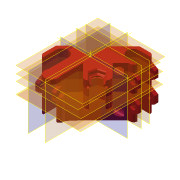
# Autodesk Inventor part: Cycl_carroX
Saved by Autodesk Inventor 2015 SP2 (Build 190223200, 223)
## iProperties
Created: 2015-05-05
Material: Genérico
Document SubType Name: Modeling
Designer: E.Beroiz
Density: 1 g/cm^3
Appearance: Light Red
Description: Cycl_carroX
Author: E.Beroiz
Autodesk Inventor part; units mm, degrees
sketch "Boceto1" plane through (0, 0, 0) normal (0, 0, 1) x (1, 0, 0)
  line L0 (0, 0) -> (0, 20)
  line L1 (0, 20) -> (17.4688, 37.4774)
  line L2 (17.4688, 37.4774) -> (29.4688, 37.4774)
  arc A0 (33.4688, 33.4774) -> (29.4688, 37.4774) centre (29.4688, 33.4774) ccw
  line L3 (33.4688, 33.4774) -> (21.7203, 33.4774)
  arc A1 (21.7203, 33.4774) -> (21.7203, 19.1774) centre (21.7203, 26.3274) ccw
  line L4 (21.7203, 19.1774) -> (33.4688, 19.1774)
  arc A2 (29.4688, 15.1774) -> (33.4688, 19.1774) centre (29.4688, 19.1774) ccw
  line L5 (29.4688, 15.1774) -> (27.2204, 15.1774)
  line L6 (27.2204, 15.1774) -> (18.5336, 6.4864)
  line L7 (18.5336, 6.4864) -> (31.5759, -6.5494)
  arc A3 (31.5778, -14.4125) -> (31.5759, -6.5494) centre (27.6454, -10.4819) ccw
  line L8 (31.5778, -14.4125) -> (23.3026, -6.1413)
  line L9 (23.3026, -6.1413) -> (15.9976, -8.1007)
  line L10 (15.9976, -8.1007) -> (14.0418, -15.4067)
  line L11 (14.0418, -15.4067) -> (22.317, -23.6778)
  arc A4 (15.7833, -23.6794) -> (22.317, -23.6778) centre (19.0494, -20.4118) ccw
  line L12 (15.7833, -23.6794) -> (2.0762, -9.9791)
  line L13 (2.0762, -9.9791) -> (2.0762, -34.9791)
  arc A5 (-11.2738, -34.9791) -> (2.0762, -34.9791) centre (-4.5988, -38.3988) ccw
  line L14 (-11.2738, -34.9791) -> (-11.2738, -13.0246)
  arc A6 (-11.2738, -13.0246) -> (-25.5738, -13.0246) centre (-18.4238, -13.0246) ccw
  line L15 (-25.5738, -13.0246) -> (-25.5738, -26.5746)
  arc A7 (-29.5738, -22.5746) -> (-25.5738, -26.5746) centre (-25.5738, -22.5746) ccw
  line L16 (-29.5738, -22.5746) -> (-29.5738, -8.5746)
  line L17 (-29.5738, -8.5746) -> (-21, 0)
  line L18 (-21, 0) -> (0, 0)
  circle A8 centre (21.3255, -13.4245) radius 4 projected
  dimension "d0" = 20
  dimension "d3" = 16
  dimension "d7" = 4
  dimension "d8" = 4
  dimension "d10" = 5.56
  dimension "d11" = 4.62
  dimension "d12" = 13.1
  dimension "d13" = 11.7
  dimension "d14" = 11.7
  dimension "d15" = 24
  dimension "d16" = 24
  dimension "d17" = 120
  dimension "d18" = 0
  dimension "d19" = 25
  dimension "d21" = 7.5
  dimension "d23" = 21
  dimension "d24" = 18
  dimension "d25" = 4
  dimension "d26" = 14.3
  dimension "d97" = 56.215
  dimension "d98" = 7.15
  dimension "d99" = 135.003
  dimension "d100" = 135.014
  dimension "d101" = 11.7485
  dimension "d102" = 2.0762
  dimension "d109" = 6.4864
  dimension "d110" = 6.551
  dimension "d111" = 6.549
  dimension "d115" = 20.5
  dimension "d116" = 19.841
  dimension "d118" = 14.3
  constraints: 38 end point, 16 point on circle, 8 centre point, 8 tangent, 7 parallel, 5 vertical, 3 horizontal alignment, 3 point on line, 2 perpendicular, 2 vertical alignment, 1 equal length, 1 horizontal
  measures "d0" distance of L0.start L0.end
  measures "d3" horizontal distance of L1.end L3.start
  measures "d7" distance between parallel lines of L3 L2
  measures "d8" distance between parallel lines of L5 L4
  measures "d10" distance between parallel lines of L7 L8
  measures "d11" distance from line of L12.start L11
  measures "d12" distance between parallel lines of L11 L8
  measures "d13" distance of L8.start L8.end
  measures "d14" distance of L10.end L11.end
  measures "d15" distance from line of L8.start L6
  measures "d16" distance from line of L11.end L6
  measures "d17" angle of L10 L9
  measures "d18" distance from line of L12.end L6
  measures "d19" distance of L12.end L13.end
  measures "d21" radius of A5
  measures "d23" distance of L17.end L0.start
  measures "d24" vertical distance of L16.end L15.end
  measures "d25" distance between parallel lines of L15 L16
  measures "d26" distance between parallel lines of L15 L14
  measures "d97" distance of A1.centre A6.centre
  measures "d98" radius of A6
  measures "d99" angle of L17 L16
  measures "d100" angle of L0 L1
  measures "d101" distance of L4.start L4.end
  measures "d102" distance from line of L0.start L13
  measures "d109" vertical distance of L6.end L0.start
  measures "d110" distance from line of L11 A8.centre
  measures "d111" distance from line of L8 A8.centre
  measures "d115" distance from line of L13 A6.centre
  measures "d116" vertical distance of L6.end A1.centre
  measures "d118" distance between parallel lines of L4 L3
extrude "Extrusión1" add sketch "Boceto1" against normal blind 5 contours L0 L1 L2 A0 L3 A1 L4 A2 L5 L6 L7 A3 L8 L9 L10 L11 A4 L12 L13 A5 L14 A6 L15 A7 L16 L17 L18
sketch "Boceto2" plane through (0, 0, -5) normal (0, 0, -1) x (-1, 0, 0)
  line L0 (0, 0) -> (0, 20) projected
  line L1 (0, 20) -> (-17.4688, 37.4774) projected
  line L2 (-17.4688, 37.4774) -> (-29.4688, 37.4774) projected
  arc A0 (-29.4688, 37.4774) -> (-33.4688, 33.4774) centre (-29.4688, 33.4774) ccw projected
  line L3 (-33.4688, 33.4774) -> (-21.7203, 33.4774) projected
  arc A1 (-21.7203, 19.1774) -> (-21.7203, 33.4774) centre (-21.7203, 26.3274) ccw projected
  line L4 (-21.7203, 19.1774) -> (-33.4688, 19.1774) projected
  arc A2 (-33.4688, 19.1774) -> (-29.4688, 15.1774) centre (-29.4688, 19.1774) ccw projected
  line L5 (-29.4688, 15.1774) -> (-27.2204, 15.1774) projected
  line L6 (-27.2204, 15.1774) -> (-18.5336, 6.4864) projected
  line L7 (-18.5336, 6.4864) -> (-31.5759, -6.5494) projected
  arc A3 (-31.5759, -6.5494) -> (-31.5778, -14.4125) centre (-27.6454, -10.4819) ccw projected
  line L8 (-31.5778, -14.4125) -> (-23.3026, -6.1413) projected
  line L9 (-23.3026, -6.1413) -> (-15.9976, -8.1007) projected
  line L10 (-15.9976, -8.1007) -> (-14.0418, -15.4067) projected
  line L11 (-14.0418, -15.4067) -> (-22.317, -23.6778) projected
  arc A4 (-22.317, -23.6778) -> (-15.7833, -23.6794) centre (-19.0494, -20.4118) ccw projected
  line L12 (-15.7833, -23.6794) -> (-2.0762, -9.9791) projected
  line L13 (-2.0762, -9.9791) -> (-2.0762, -34.9791) projected
  arc A5 (-2.0762, -34.9791) -> (11.2738, -34.9791) centre (4.5988, -38.3988) ccw projected
  line L14 (11.2738, -34.9791) -> (11.2738, -13.0246) projected
  arc A6 (25.5738, -13.0246) -> (11.2738, -13.0246) centre (18.4238, -13.0246) ccw projected
  line L15 (25.5738, -13.0246) -> (25.5738, -26.5746) projected
  arc A7 (25.5738, -26.5746) -> (29.5738, -22.5746) centre (25.5738, -22.5746) ccw projected
  line L16 (29.5738, -22.5746) -> (29.5738, -8.5746) projected
  line L17 (29.5738, -8.5746) -> (21, 0) projected
  line L18 (21, 0) -> (0, 0) projected
  line L19 (-2.0762, -9.9791) -> (7.2738, -20.5746)
  line L20 (7.2738, -20.5746) -> (7.2738, -22.5746)
  arc A8 (7.2738, -22.5746) -> (11.2738, -26.5746) centre (11.2738, -22.5746) ccw
  dimension "d30" = 4
  dimension "d31" = 2
  constraints: 4 end point, 2 horizontal alignment, 2 point on circle, 1 centre point, 1 point on line, 1 tangent, 1 vertical, 1 vertical alignment
  measures "d30" distance between parallel lines of L14 L20
  measures "d31" distance of L19.end L20.end
extrude "Extrusión2" add sketch "Boceto2" along normal blind 25.5 contours L18 L17 L16 A7 L15 A6 L14 A8 L20 L19 L12 A4 L11 L10 L9 L8 A3 L7 L6 L5 A2 L4 A1 L3 A0 L2 L1 L0
sketch "Boceto3" plane through (0, 0, -30.5) normal (0, 0, -1) x (-1, 0, 0)
  line L0 (0, 0) -> (0, 20) projected
  line L1 (0, 20) -> (-17.4688, 37.4774) projected
  line L2 (-17.4688, 37.4774) -> (-29.4688, 37.4774) projected
  arc A0 (-29.4688, 37.4774) -> (-33.4688, 33.4774) centre (-29.4688, 33.4774) ccw projected
  line L3 (-33.4688, 33.4774) -> (-21.7203, 33.4774) projected
  arc A1 (-21.7203, 19.1774) -> (-21.7203, 33.4774) centre (-21.7203, 26.3274) ccw projected
  line L4 (-21.7203, 19.1774) -> (-33.4688, 19.1774) projected
  arc A2 (-33.4688, 19.1774) -> (-29.4688, 15.1774) centre (-29.4688, 19.1774) ccw projected
  line L5 (-29.4688, 15.1774) -> (-27.2204, 15.1774) projected
  line L6 (-27.2204, 15.1774) -> (-18.5336, 6.4864) projected
  line L7 (-18.5336, 6.4864) -> (-31.5759, -6.5494) projected
  arc A3 (-31.5759, -6.5494) -> (-31.5778, -14.4125) centre (-27.6454, -10.4819) ccw projected
  line L8 (-31.5778, -14.4125) -> (-23.3026, -6.1413) projected
  line L9 (-23.3026, -6.1413) -> (-15.9976, -8.1007) projected
  line L10 (-15.9976, -8.1007) -> (-14.0418, -15.4067) projected
  line L11 (-14.0418, -15.4067) -> (-22.317, -23.6778) projected
  arc A4 (-22.317, -23.6778) -> (-15.7833, -23.6794) centre (-19.0494, -20.4118) ccw projected
  line L12 (-15.7833, -23.6794) -> (-2.0762, -9.9791) projected
  line L13 (-2.0762, -9.9791) -> (7.2738, -20.5746) projected
  line L14 (7.2738, -20.5746) -> (7.2738, -22.5746) projected
  arc A5 (7.2738, -22.5746) -> (11.2738, -26.5746) centre (11.2738, -22.5746) ccw projected
  line L15 (11.2738, -26.5746) -> (11.2738, -13.0246) projected
  arc A6 (25.5738, -13.0246) -> (11.2738, -13.0246) centre (18.4238, -13.0246) ccw projected
  line L16 (25.5738, -13.0246) -> (25.5738, -26.5746) projected
  arc A7 (25.5738, -26.5746) -> (29.5738, -22.5746) centre (25.5738, -22.5746) ccw projected
  line L17 (29.5738, -22.5746) -> (29.5738, -8.5746) projected
  line L18 (29.5738, -8.5746) -> (21, 0) projected
  line L19 (21, 0) -> (0, 0) projected
  line L20 (-18.5336, 6.4864) -> (-2.0762, -9.9791)
  constraints: 2 end point
extrude "Extrusión3" add sketch "Boceto3" along normal blind 25 contours L19 L18 L17 A7 L16 A6 L15 A5 L14 L13 L20 L6 L5 A2 L4 A1 L3 A0 L2 L1 L0
sketch "Boceto4" plane through (-29.5738, -22.5746, 0) normal (-1, 0, 0) x (0, 0, 1)
  line L0 (0, 0) -> (0, 14) projected
  line L1 (0, 14) -> (-55.5, 14) projected
  line L2 (-55.5, 0) -> (-55.5, 14) projected
  line L3 (0, 0) -> (-55.5, 0) projected
  line L4 (0, 14) -> (-55.5, 14) projected
  line L5 (-5.75, 14) -> (-20.8896, 28.2756)
  arc A0 (-20.8896, 28.2756) -> (-34.6104, 28.2756) centre (-27.75, 21) ccw
  line L6 (-34.6104, 28.2756) -> (-49.75, 14)
  line L7 (0, -4) -> (-55.5, -4) projected
  point P0 (0, 22.5746)
  point P1 (-27.75, 0)
  dimension "d36" = 25
  dimension "d37" = 44
  dimension "d38" = 10
  constraints: 4 end point, 2 point on circle, 2 point on line, 2 tangent, 1 centre point, 1 equal length, 1 midpoint, 1 vertical alignment
  measures "d36" distance from line of L7 A0.centre
  measures "d37" distance of L6.end L5.start
  measures "d38" radius of A0
extrude "Extrusión4" add sketch "Boceto4" against normal blind 10 contours L1 L6 A0 L5
ref_plane "Plano de trabajo1" through (0, 0, -27.75) normal (0, 0, 1) x (1, 0, 0)
sketch "Boceto7" plane through (0, 0, -27.75) normal (0, 0, 1) x (1, 0, 0)
  arc A0 (-19.5738, -5.9677) -> (-24.0202, -8.5746) centre (-18.4238, -13.0246) ccw projected
  line L0 (-19.5738, -8.5746) -> (-19.5738, -5.9677) projected
  line L1 (-24.0202, -8.5746) -> (-19.5738, -8.5746) projected
  point P0 (0, 0)
extrude "Extrusión8" cut sketch "Boceto7" along normal through all both and the other way through all
sketch "Boceto8" plane through (-29.5738, -22.5746, 0) normal (-1, 0, 0) x (0, 0, 1)
  line L0 (-20.0135, 21.425) -> (-23.8818, 14.725)
  line L1 (-23.8818, 14.725) -> (-31.6182, 14.725)
  line L2 (-31.6182, 14.725) -> (-35.4865, 21.425)
  line L3 (-35.4865, 21.425) -> (-31.6182, 28.125)
  line L4 (-31.6182, 28.125) -> (-23.8818, 28.125)
  line L5 (-23.8818, 28.125) -> (-20.0135, 21.425)
  arc A0 (-20.8896, 28.2756) -> (-34.6104, 28.2756) centre (-27.75, 21) ccw projected
  point P0 (0, 22.5746)
  point P1 (-27.75, 31)
  point P2 (-27.75, 28.125)
  point P3 (-27.75, 14.725)
  dimension "d50" = 13.4
  dimension "d112" = 120
  dimension "d113" = 120
  dimension "d114" = 0.425
  constraints: 12 end point, 5 equal length, 2 midpoint, 2 vertical alignment, 1 point on circle
  measures "d50" distance between parallel lines of L4 L1
  measures "d112" angle of L0 L5
  measures "d113" angle of L5 L4
  measures "d114" vertical distance of L0.start A0.centre
extrude "Extrusión9" cut sketch "Boceto8" against normal blind 5.5
sketch "Boceto9" plane through (-19.5738, -22.5746, 0) normal (1, 0, 0) x (0, 0, -1)
  line L0 (20.0135, 21.425) -> (23.8818, 14.725) projected
  line L1 (23.8818, 28.125) -> (20.0135, 21.425) projected
  line L2 (31.6182, 28.125) -> (23.8818, 28.125) projected
  line L3 (35.4865, 21.425) -> (31.6182, 28.125) projected
  line L4 (31.6182, 14.725) -> (35.4865, 21.425) projected
  line L5 (31.6182, 14.925) -> (23.8818, 14.925) projected
  circle A0 centre (27.75, 21.4246) radius 4.5
  point P0 (0, 22.5746)
  dimension "d53" = 9
  constraints: 1 centre point
  measures "d53" diameter of A0
extrude "Extrusión10" add sketch "Boceto9" against normal blind 3.5
sketch "Boceto10" plane through (0, 0, 0) normal (-1, 0, 0) x (0, 0, 1)
  line L0 (0, 0) -> (-55.5, 0) projected
  line L1 (0, 0) -> (0, 20) projected
  line L2 (0, 20) -> (-55.5, 20) projected
  line L3 (-55.5, 0) -> (-55.5, 20) projected
  circle A0 centre (-7.75, 11) radius 4.15
  circle A1 centre (-47.75, 11) radius 4.15
  dimension "d56" = 8.3
  dimension "d57" = 8.3
  dimension "d58" = 40
  dimension "d59" = 7.75
  dimension "d60" = 11
  constraints: 2 centre point, 1 horizontal alignment
  measures "d56" diameter of A0
  measures "d57" diameter of A1
  measures "d58" distance of A1.centre A0.centre
  measures "d59" distance from line of L3 A1.centre
  measures "d60" distance from line of L0 A0.centre
extrude "Extrusión11" cut sketch "Boceto10" against normal blind 25 contours A0 | A1
sketch "Boceto11" plane through (-29.5738, -22.5746, 0) normal (-1, 0, 0) x (0, 0, 1)
  line L0 (-23.8818, 28.125) -> (-20.0135, 21.425) projected
  line L1 (-20.0135, 21.425) -> (-23.8818, 14.725) projected
  line L2 (-23.8818, 14.725) -> (-31.6182, 14.725) projected
  line L3 (-31.6182, 14.725) -> (-35.4865, 21.425) projected
  line L4 (-35.4865, 21.425) -> (-31.6182, 28.125) projected
  line L5 (-31.6182, 28.125) -> (-23.8818, 28.125) projected
  line L6 (0, 0) -> (0, 14) projected
  line L7 (0, 14) -> (-5.75, 14) projected
  line L8 (-5.75, 14) -> (-20.8896, 28.2756) projected
  arc A0 (-20.8896, 28.2756) -> (-34.6104, 28.2756) centre (-27.75, 21) ccw projected
  line L9 (-34.6104, 28.2756) -> (-49.75, 14) projected
  line L10 (-49.75, 14) -> (-55.5, 14) projected
  line L11 (-55.5, 0) -> (-55.5, 14) projected
  line L12 (0, 0) -> (-55.5, 0) projected
  line L13 (-24.75, -7) -> (-30.75, -7)
  line L14 (-30.75, -7) -> (-33.75, -1.8038)
  line L15 (-33.75, -1.8038) -> (-30.75, 3.3923)
  line L16 (-30.75, 3.3923) -> (-24.75, 3.3923)
  line L17 (-24.75, 3.3923) -> (-21.75, -1.8038)
  line L18 (-21.75, -1.8038) -> (-24.75, -7)
  line L19 (0, -4) -> (-55.5, -4) projected
  point P0 (0, 22.5746)
  point P1 (-27.75, -1.8038)
  dimension "d63" = 3
  dimension "d64" = 6
  constraints: 12 end point, 1 horizontal, 1 vertical alignment, 13 other
  measures "d63" distance between parallel lines of L13 L19
  measures "d64" distance of L13.start L13.end
extrude "Extrusión12" add sketch "Boceto11" against normal up to surface (4 mm away) contours L17 L18 L19 L14 L15 L12 | L12 L15 L16 L17 | L18 L13 L14 L19
sketch "Boceto12" plane through (-29.5738, -22.5746, 0) normal (-1, 0, 0) x (0, 0, 1)
  line L0 (0, 0) -> (-22.7915, 0) projected
  line L1 (0, 0) -> (0, 14) projected
  line L2 (0, 14) -> (-5.75, 14) projected
  line L3 (-5.75, 14) -> (-20.8896, 28.2756) projected
  arc A0 (-20.8896, 28.2756) -> (-34.6104, 28.2756) centre (-27.75, 21) ccw projected
  line L4 (-34.6104, 28.2756) -> (-49.75, 14) projected
  line L5 (-49.75, 14) -> (-55.5, 14) projected
  line L6 (-55.5, 0) -> (-55.5, 14) projected
  line L7 (-32.7085, 0) -> (-55.5, 0) projected
  line L8 (-33.75, -1.8038) -> (-32.7085, 0) projected
  line L9 (-30.75, -7) -> (-33.75, -1.8038) projected
  line L10 (-24.75, -7) -> (-30.75, -7) projected
  line L11 (-21.75, -1.8038) -> (-24.75, -7) projected
  line L12 (-22.7915, 0) -> (-21.75, -1.8038) projected
  line L13 (-23.8818, 28.125) -> (-20.0135, 21.425) projected
  line L14 (-20.0135, 21.425) -> (-23.8818, 14.725) projected
  line L15 (-23.8818, 14.725) -> (-31.6182, 14.725) projected
  line L16 (-31.6182, 14.725) -> (-35.4865, 21.425) projected
  line L17 (-35.4865, 21.425) -> (-31.6182, 28.125) projected
  line L18 (-31.6182, 28.125) -> (-23.8818, 28.125) projected
  circle A1 centre (-27.75, -1.8038) radius 3.5
  point P0 (0, 22.5746)
  point P1 (-27.75, -7)
  dimension "d67" = 7
  constraints: 1 centre point, 1 horizontal alignment, 1 midpoint, 1 vertical alignment
  measures "d67" diameter of A1
extrude "Extrusión13" cut sketch "Boceto12" against normal blind 2 contours A1
sketch "Boceto13" plane through (-27.5738, -24.3785, -27.75) normal (-1, 0, 0) x (0, 0, 1)
  circle A0 centre (0, 0) radius 3.5 projected
  circle A1 centre (0, 0) radius 1.875
  point P0 (27.75, 24.3785)
  dimension "d70" = 3.75
  constraints: 1 centre point, 1 coincident
  measures "d70" diameter of A1
extrude "Extrusión14" cut sketch "Boceto13" against normal up to surface (2 mm away) contours A1
ref_plane "Plano de trabajo2" through (-18.4238, -34.9791, 0) normal (-1, 0, 0) x (0, 0, 1)
mirror "Simetría1" about plane through (-18.4238, -34.9791, 0) normal (-1, 0, 0) of "Extrusión12"
sketch "Boceto14" plane through (-7.2738, -22.5746, -5) normal (1, 0, 0) x (0, 0, -1)
  line L0 (20.9501, -4.9213) -> (19.1502, -1.8038)
  line L1 (19.1502, -1.8038) -> (20.9501, 1.3137)
  line L2 (20.9501, 1.3137) -> (24.5499, 1.3137)
  line L3 (24.5499, 1.3137) -> (26.3498, -1.8038)
  line L4 (26.3498, -1.8038) -> (24.5499, -4.9213)
  line L5 (24.5499, -4.9213) -> (20.9501, -4.9213)
  line L6 (19.75, -7) -> (25.75, -7) projected
  circle A0 centre (22.75, -1.8038) radius 1.875 projected
  line L7 (27.4821, -4) -> (50.5, -4) projected
  line L8 (50.5, 9.55) -> (50.5, -4) projected
  line L9 (-5, 9.55) -> (50.5, 9.55) projected
  line L10 (-5, 9.55) -> (-5, -4) projected
  line L11 (-5, -4) -> (18.0179, -4) projected
  line L12 (19.75, -7) -> (18.0179, -4) projected
  line L13 (25.75, -7) -> (19.75, -7) projected
  line L14 (27.4821, -4) -> (25.75, -7) projected
  point P0 (-5, 22.5746)
  point P1 (22.75, -1.8038)
  point P2 (22.75, -7)
  dimension "d73" = 6.235
  constraints: 12 end point, 1 coincident, 1 horizontal, 1 midpoint, 1 vertical alignment, 13 other
  measures "d73" distance between parallel lines of L5 L2
extrude "Extrusión15" cut sketch "Boceto14" against normal blind 3 contours L0 L1 L2 L3 L4 L5 | A0
sketch "Boceto15" plane through (-10.2738, -22.5746, -5) normal (1, 0, 0) x (0, 0, -1)
  circle A0 centre (22.75, -1.8038) radius 1.875 projected
  point P0 (-5, 22.5746)
extrude "Extrusión16" cut sketch "Boceto15" against normal blind 3
sketch "Boceto16" plane through (17.4688, 37.4774, 0) normal (0, 1, 0) x (1, 0, 0)
  line L0 (0, 0) -> (12, 0) projected
  line L1 (12, 0) -> (12, 55.5) projected
  line L2 (0, 55.5) -> (12, 55.5) projected
  line L3 (0, 0) -> (0, 55.5) projected
  line L4 (16, 0) -> (16, 55.5) projected
  line L5 (14, 7.6671) -> (7, 11.7085)
  line L6 (7, 11.7085) -> (7, 19.7915)
  line L7 (7, 19.7915) -> (14, 23.8329)
  line L8 (14, 23.8329) -> (21, 19.7915)
  line L9 (21, 19.7915) -> (21, 11.7085)
  line L10 (21, 11.7085) -> (14, 7.6671)
  line L11 (14, 31.6671) -> (7, 35.7085)
  line L12 (7, 35.7085) -> (7, 43.7915)
  line L13 (7, 43.7915) -> (14, 47.8329)
  line L14 (14, 47.8329) -> (21, 43.7915)
  line L15 (21, 43.7915) -> (21, 35.7085)
  line L16 (21, 35.7085) -> (14, 31.6671)
  line L17 (16, 0) -> (12, 0) projected
  point P0 (-17.4688, 0)
  point P1 (14, 15.75)
  point P2 (14, 39.75)
  dimension "d78" = 24
  dimension "d79" = 14
  dimension "d80" = 15.75
  dimension "d81" = 2
  constraints: 24 end point, 2 vertical, 2 vertical alignment, 26 other
  measures "d78" distance of point (14, 39.75) point (14, 15.75)
  measures "d79" distance from line of L6 L8.end
  measures "d80" distance from line of L17 point (14, 15.75)
  measures "d81" distance from line of L4 point (14, 15.75)
extrude "Extrusión17" add sketch "Boceto16" against normal up to surface (4 mm away) contours L5 L6 L7 L1 | L1 L7 L8 L4 L10 L5 | L4 L8 L9 L10 | L13 L14 L4 L16 L11 L1 | L1 L11 L12 L13 | L4 L14 L15 L16
ref_plane "Plano de trabajo3" through (21.7203, 26.3274, 0) normal (0, -1, 0) x (1, 0, 0)
mirror "Simetría2" about plane through (21.7203, 26.3274, 0) normal (0, -1, 0) of "Extrusión17"
ref_plane "Plano de trabajo4" through (0, 0, -27.75) normal (0, 0, 1) x (1, 0, 0)
sketch "Boceto17" plane through (17.4688, 37.4774, 0) normal (0, 1, 0) x (1, 0, 0)
  line L0 (12, 46.6782) -> (12, 55.5) projected
  line L1 (0, 55.5) -> (12, 55.5) projected
  line L2 (0, 0) -> (0, 55.5) projected
  line L3 (0, 0) -> (12, 0) projected
  line L4 (12, 0) -> (12, 8.8218) projected
  line L5 (14, 7.6671) -> (12, 8.8218) projected
  line L6 (21, 11.7085) -> (14, 7.6671) projected
  line L7 (21, 19.7915) -> (21, 11.7085) projected
  line L8 (14, 23.8329) -> (21, 19.7915) projected
  line L9 (12, 22.6782) -> (14, 23.8329) projected
  line L10 (12, 22.6782) -> (12, 32.8218) projected
  line L11 (14, 31.6671) -> (12, 32.8218) projected
  line L12 (21, 35.7085) -> (14, 31.6671) projected
  line L13 (21, 43.7915) -> (21, 35.7085) projected
  line L14 (14, 47.8329) -> (21, 43.7915) projected
  line L15 (12, 46.6782) -> (14, 47.8329) projected
  circle A0 centre (14.6667, 15.75) radius 3.5
  circle A1 centre (14.6667, 39.75) radius 3.5
  point P0 (-17.4688, 0)
  dimension "d84" = 7
  dimension "d85" = 7
  constraints: 2 centre point
  measures "d84" diameter of A0
  measures "d85" diameter of A1
extrude "Extrusión18" cut sketch "Boceto17" against normal blind 2 contours A0 | A1
sketch "Boceto18" plane through (32.1355, 35.4774, -15.75) normal (0, 1, 0) x (1, 0, 0)
  circle A0 centre (0, 0) radius 3.5 projected
  circle A1 centre (0, 24) radius 3.5 projected
  circle A2 centre (0, 0) radius 1.875
  circle A3 centre (0, 24) radius 1.875
  point P0 (-32.1355, -15.75)
  dimension "d88" = 3.75
  dimension "d89" = 3.75
  constraints: 2 centre point, 2 coincident
  measures "d88" diameter of A2
  measures "d89" diameter of A3
extrude "Extrusión19" cut sketch "Boceto18" against normal blind 30 contours A2 | A3
ref_plane "Plano de trabajo5" through (27.2204, 17.1774, 0) normal (0, -1, 0) x (1, 0, 0)
sketch "Boceto19" plane through (27.2204, 15.1774, 0) normal (0, -1, 0) x (1, 0, 0)
  circle A0 centre (4.9151, -39.75) radius 1.875 projected
  circle A1 centre (4.9151, -15.75) radius 1.875 projected
  line L0 (8.0326, -37.9501) -> (8.0326, -41.5499)
  line L1 (8.0326, -41.5499) -> (4.9151, -43.3498)
  line L2 (4.9151, -43.3498) -> (1.7976, -41.5499)
  line L3 (1.7976, -41.5499) -> (1.7976, -37.9501)
  line L4 (1.7976, -37.9501) -> (4.9151, -36.1502)
  line L5 (4.9151, -36.1502) -> (8.0326, -37.9501)
  line L6 (8.0326, -13.9501) -> (8.0326, -17.5499)
  line L7 (8.0326, -17.5499) -> (4.9151, -19.3498)
  line L8 (4.9151, -19.3498) -> (1.7976, -17.5499)
  line L9 (1.7976, -17.5499) -> (1.7976, -13.9501)
  line L10 (1.7976, -13.9501) -> (4.9151, -12.1502)
  line L11 (4.9151, -12.1502) -> (8.0326, -13.9501)
  point P0 (-27.2204, 0)
  dimension "d92" = 6.235
  dimension "d93" = 6.235
  constraints: 24 end point, 2 coincident, 2 vertical, 26 other
  measures "d92" distance between parallel lines of L4 L1
  measures "d93" distance between parallel lines of L10 L7
extrude "Extrusión20" cut sketch "Boceto19" against normal blind 2.8
sketch "Boceto20" plane through (0, 0, -27.75) normal (0, 0, 1) x (1, 0, 0)
  arc A0 (-11.2738, -13.0246) -> (-25.5738, -13.0246) centre (-18.4238, -13.0246) ccw projected
  circle A1 centre (-18.4238, -13.0246) radius 7.55
  point P0 (0, 0)
  dimension "d103" = 15.1
  constraints: 1 centre point, 1 coincident
  measures "d103" diameter of A1
extrude "Extrusión21" cut sketch "Boceto20" along normal mid plane 24.2
sketch "Boceto21" plane through (0, 0, -27.75) normal (0, 0, 1) x (1, 0, 0)
  arc A0 (21.7203, 33.4774) -> (21.7203, 19.1774) centre (21.7203, 26.3274) ccw projected
  circle A1 centre (21.7203, 26.3274) radius 7.55
  point P0 (0, 0)
  dimension "d106" = 15.1
  constraints: 1 centre point, 1 coincident
  measures "d106" diameter of A1
extrude "Extrusión22" cut sketch "Boceto21" along normal mid plane 48.4
ref_plane "Plano de trabajo6" through (0, 0, -15.25) normal (0, 0, 1) x (1, 0, 0)
ref_plane "Plano de trabajo7" through (0, 0, -8) normal (0, 0, 1) x (1, 0, 0)
sketch "Boceto26" plane through (0, 0, -8) normal (0, 0, 1) x (1, 0, 0)
  line L0 (15.9976, -8.1007) -> (14.0418, -15.4067) projected
  line L1 (14.0418, -15.4067) -> (22.317, -23.6778) projected
  line L2 (23.3026, -6.1413) -> (15.9976, -8.1007) projected
  line L3 (31.5778, -14.4125) -> (23.3026, -6.1413) projected
  line L4 (23.3026, -6.1413) -> (24.3114, -7.1496) projected
  line L5 (15.9976, -8.1007) -> (23.3026, -6.1413)
  line L6 (23.3026, -6.1413) -> (28.652, -11.4881)
  line L7 (28.652, -11.4881) -> (26.6963, -18.7941)
  line L8 (26.6963, -18.7941) -> (19.3912, -20.7535)
  line L9 (19.3912, -20.7535) -> (14.0418, -15.4067)
  line L10 (14.0418, -15.4067) -> (15.9976, -8.1007)
  arc A0 (27.6421, -8.1928) -> (15.5501, -19.2471) centre (21.3469, -13.4474) ccw
  line L11 (22.101, -25.7948) -> (33.6712, -14.219)
  line L12 (33.6712, -14.219) -> (26.5984, -7.1496)
  line L13 (22.101, -25.7948) -> (15.5501, -19.2471)
  point P0 (0, 0)
  point P1 (19.5434, -7.1496)
  dimension "d128" = 16.4
  dimension "d129" = 10
  constraints: 18 end point, 3 point on circle, 2 parallel, 1 centre point, 1 coincident, 1 collinear, 1 perpendicular, 1 point on line, 1 tangent, 13 other
  measures "d128" diameter of A0
  measures "d129" distance of L11.end L12.end
extrude "Extrusión27" cut sketch "Boceto26" along normal blind 2.2 contours L2 L3 L7 L8 L1 L0 | L12 A0 | L12 L11 L13 A0
sketch "Boceto27" plane through (0, 0, -5.8) normal (0, 0, -1) x (-1, 0, 0)
  line L0 (0, 0) -> (0, 20) projected
  line L1 (21, 0) -> (0, 0) projected
  line L2 (29.5738, -8.5746) -> (21, 0) projected
  line L3 (29.5738, -22.5746) -> (29.5738, -8.5746) projected
  arc A0 (25.5738, -26.5746) -> (29.5738, -22.5746) centre (25.5738, -22.5746) ccw projected
  line L4 (25.5738, -13.0246) -> (25.5738, -26.5746) projected
  arc A1 (25.5738, -13.0246) -> (11.2738, -13.0246) centre (18.4238, -13.0246) ccw projected
  line L5 (11.2738, -34.9791) -> (11.2738, -13.0246) projected
  arc A2 (-2.0762, -34.9791) -> (11.2738, -34.9791) centre (4.5988, -38.3988) ccw projected
  line L6 (-2.0762, -9.9791) -> (-2.0762, -34.9791) projected
  line L7 (-15.7833, -23.6794) -> (-2.0762, -9.9791) projected
  arc A3 (-22.317, -23.6778) -> (-15.7833, -23.6794) centre (-19.0494, -20.4118) ccw projected
  line L8 (-14.0418, -15.4067) -> (-22.317, -23.6778) projected
  line L9 (-15.9976, -8.1007) -> (-14.0418, -15.4067) projected
  line L10 (-23.3026, -6.1413) -> (-15.9976, -8.1007) projected
  line L11 (-31.5778, -14.4125) -> (-23.3026, -6.1413) projected
  arc A4 (-31.5759, -6.5494) -> (-31.5778, -14.4125) centre (-27.6454, -10.4819) ccw projected
  line L12 (-18.5336, 6.4864) -> (-31.5759, -6.5494) projected
  line L13 (-27.2204, 15.1774) -> (-18.5336, 6.4864) projected
  line L14 (-29.4688, 15.1774) -> (-27.2204, 15.1774) projected
  arc A5 (-33.4688, 19.1774) -> (-29.4688, 15.1774) centre (-29.4688, 19.1774) ccw projected
  line L15 (-21.7203, 19.1774) -> (-33.4688, 19.1774) projected
  arc A6 (-21.7203, 19.1774) -> (-21.7203, 33.4774) centre (-21.7203, 26.3274) ccw projected
  line L16 (-33.4688, 33.4774) -> (-21.7203, 33.4774) projected
  arc A7 (-29.4688, 37.4774) -> (-33.4688, 33.4774) centre (-29.4688, 33.4774) ccw projected
  line L17 (-17.4688, 37.4774) -> (-29.4688, 37.4774) projected
  line L18 (0, 20) -> (-17.4688, 37.4774) projected
  line L19 (-30.4821, -15.5087) -> (-24.8816, -9.911)
  arc A8 (-17.8123, -16.9838) -> (-24.8816, -9.911) centre (-21.3469, -13.4474) ccw
  line L20 (-17.8123, -16.9838) -> (-23.4128, -22.5816)
  line L21 (-23.4128, -22.5816) -> (-22.317, -23.6778)
  line L22 (-14.0418, -15.4067) -> (-22.317, -23.6778)
  line L23 (-22.317, -23.6778) -> (-14.0418, -15.4067)
  line L24 (-14.0418, -15.4067) -> (-22.317, -23.6778) projected
  line L25 (-15.9976, -8.1007) -> (-23.3026, -6.1413)
  line L26 (-23.3026, -6.1413) -> (-31.5778, -14.4125)
  line L27 (-31.5778, -14.4125) -> (-23.3026, -6.1413) projected
  line L28 (-31.5778, -14.4125) -> (-23.3026, -6.1413)
  line L29 (-31.5778, -14.4125) -> (-30.4821, -15.5087)
  line L30 (-15.9976, -8.1007) -> (-14.0418, -15.4067)
  line L31 (-14.0418, -15.4067) -> (-19.3912, -20.7535)
  line L32 (-28.652, -11.4881) -> (-23.3026, -6.1413)
  line L33 (-23.3026, -6.1413) -> (-15.9976, -8.1007)
  dimension "d132" = 5
  constraints: 26 end point, 6 collinear, 3 parallel, 2 equal length, 2 perpendicular, 2 point on circle, 2 tangent, 1 centre point, 1 coincident, 8 other
  measures "d132" radius of A8
extrude "Extrusión28" add sketch "Boceto27" against normal blind 1.5 contours L21 L20 A8 L19 L29 L11 L10 L9 L8
fillet "Empalme1" radius 0.5 6 edges at (17.8105, -9.9127, -4.3) (27.6818, -12.7099, -4.3) (20.6125, -19.7827, -4.3) (17.8105, -9.9127, -5.8) (27.6818, -12.7099, -5.8) (20.6125, -19.7827, -5.8)
chamfer "Chaflán1" distance 1 angle 45 4 edges at (18.1794, -19.5423, -4.3) (15.0197, -11.7537, -4.3) (19.6501, -7.121, -4.3) (27.4402, -10.2769, -4.3)
chamfer "Chaflán2" distance 1.5 angle 30 1 edges at (0, 11, -11.9) measured on face at (16.2727, 12.2527, -11.7064)
chamfer "Chaflán3" distance 1.5 angle 30 1 edges at (0, 11, -51.9) measured on face at (16.2727, 12.2527, -51.7064)
sketch "Boceto28" plane through (-7.2738, -22.5746, -5) normal (1, 0, 0) x (0, 0, -1)
  line L0 (17.7915, 0) -> (16.75, -1.8038) projected
  line L1 (16.75, -1.8038) -> (18.0179, -4) projected
  line L2 (19.75, -7) -> (18.0179, -4) projected
  line L3 (25.75, -7) -> (19.75, -7) projected
  line L4 (27.4821, -4) -> (25.75, -7) projected
  line L5 (27.4821, -4) -> (28.75, -1.8038) projected
  line L6 (28.75, -1.8038) -> (27.7085, 0) projected
  line L7 (28.0179, 3.4641) -> (31.0594, -1.8038)
  line L8 (31.0594, -1.8038) -> (29.2141, -5)
  line L9 (29.2141, -5) -> (26.9047, -9)
  line L10 (26.9047, -9) -> (18.5953, -9)
  line L11 (18.5953, -9) -> (16.2859, -5)
  line L12 (16.2859, -5) -> (14.4406, -1.8038)
  line L13 (14.4406, -1.8038) -> (17.4821, 3.4641)
  line L14 (17.4821, 3.4641) -> (22.75, 6.5056)
  line L15 (22.75, 6.5056) -> (28.0179, 3.4641)
  circle A0 centre (22.75, -1.8038) radius 1.875 projected
  line L16 (20.9501, -4.9213) -> (19.1502, -1.8038) projected
  line L17 (24.5499, -4.9213) -> (20.9501, -4.9213) projected
  line L18 (26.3498, -1.8038) -> (24.5499, -4.9213) projected
  line L19 (24.5499, 1.3137) -> (26.3498, -1.8038) projected
  line L20 (20.9501, 1.3137) -> (24.5499, 1.3137) projected
  line L21 (19.1502, -1.8038) -> (20.9501, 1.3137) projected
  point P0 (-5, 22.5746)
  dimension "d145" = 2
  dimension "d146" = 120
  constraints: 18 end point, 3 equal length, 6 other
  measures "d145" distance between parallel lines of L1 L12
  measures "d146" angle of L15 L14
extrude "Extrusión29" add sketch "Boceto28" against normal up to surface (4 mm away) contours L7 L8 L9 L10 L11 L12 L13 L14 L15
sketch "Boceto29" plane through (-29.5738, -22.5746, 0) normal (-1, 0, 0) x (0, 0, 1)
  line L0 (-32.4821, -4) -> (-30.75, -7) projected
  line L1 (-30.75, -7) -> (-24.75, -7) projected
  line L2 (-24.75, -7) -> (-23.0179, -4) projected
  line L3 (-23.0179, -4) -> (-21.75, -1.8038) projected
  line L4 (-21.75, -1.8038) -> (-22.7915, 0) projected
  line L5 (-32.7085, 0) -> (-33.75, -1.8038) projected
  line L6 (-33.75, -1.8038) -> (-32.4821, -4) projected
  line L7 (-20.8865, 0.7005) -> (-19.4406, -1.8038)
  line L8 (-19.4406, -1.8038) -> (-21.2859, -5)
  line L9 (-21.2859, -5) -> (-23.5953, -9)
  line L10 (-23.5953, -9) -> (-31.9047, -9)
  line L11 (-31.9047, -9) -> (-34.2141, -5)
  line L12 (-34.2141, -5) -> (-36.0594, -1.8038)
  line L13 (-36.0594, -1.8038) -> (-34.6135, 0.7005)
  line L14 (-34.6135, 0.7005) -> (-27.75, 4.6631)
  line L15 (-27.75, 4.6631) -> (-20.8865, 0.7005)
  circle A0 centre (-27.75, -1.8038) radius 3.5 projected
  point P0 (0, 22.5746)
  point P1 (-27.75, -7)
  dimension "d149" = 2
  dimension "d152" = 120
  constraints: 18 end point, 1 equal length, 1 midpoint, 1 vertical alignment, 6 other
  measures "d149" distance between parallel lines of L6 L12
  measures "d152" angle of L15 L14
extrude "Extrusión30" add sketch "Boceto29" against normal up to surface (4 mm away)
sketch "Sketch30" plane through (-24.0738, -22.5746, 0) normal (-1, 0, 0) x (0, 0, 1)
  circle A0 centre (-27.75, 21) radius 4.5
  arc A1 (-20.8896, 28.2756) -> (-34.6104, 28.2756) centre (-27.75, 21) ccw projected
  point P0 (0, 22.5746)
  dimension "d155" = 9
  constraints: 1 centre point, 1 concentric
  measures "d155" diameter of A0
extrude "Extrusion31" cut sketch "Sketch30" against normal through all
chamfer "Chamfer4" distance 1 angle 45 4 edges at (18.1794, -19.5423, 0) (15.0197, -11.7537, 0) (19.6501, -7.121, 0) (27.4402, -10.2769, 0)
fillet "Empalme2" radius 1 4 edges at (15.0197, -11.7537, -1) (19.6501, -7.121, -1) (27.4402, -10.2769, -1) (18.1794, -19.5423, -1)
